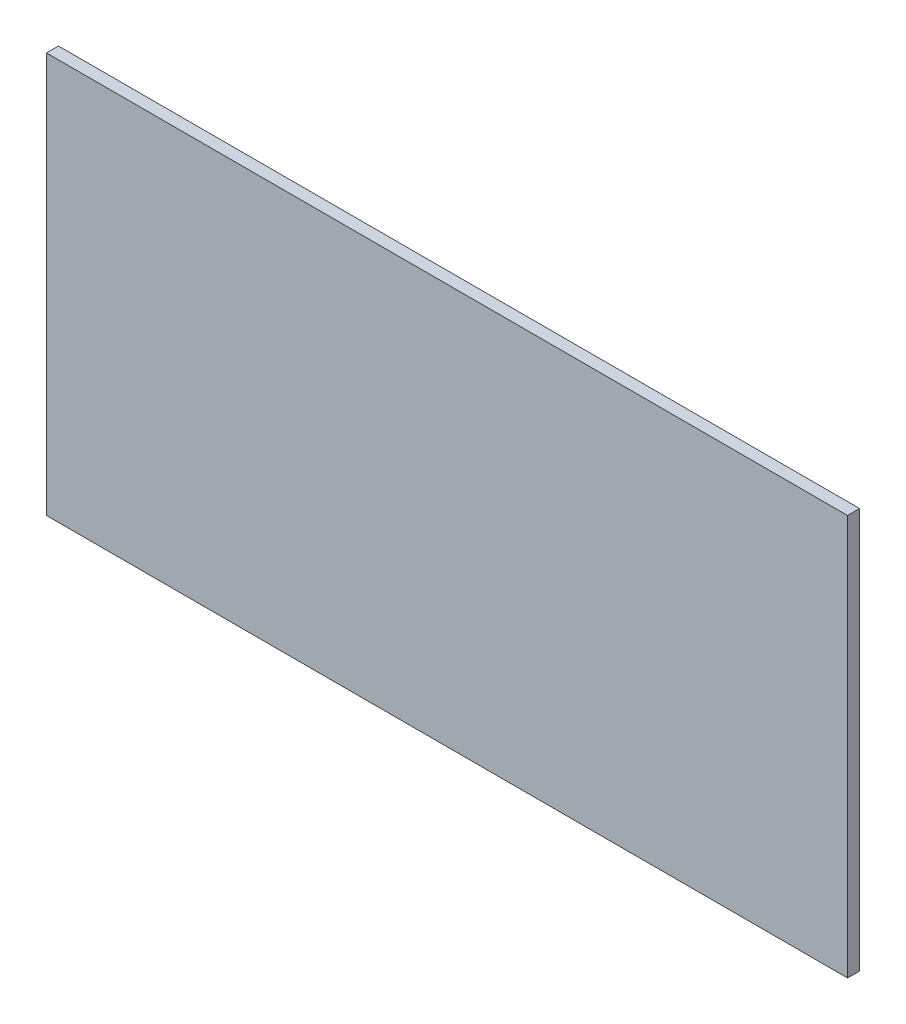
# Autodesk Inventor part: 받침
Saved by Autodesk Inventor 2016 (Build 200138000, 138)
## iProperties
Created: 2024-03-15
Part Number: 받침
Material: 카펫
Document SubType Name: Modeling
Designer: pc
Density: 0.19 g/cm^3
Appearance: 섬세 - 흰색
Author: pc
Autodesk Inventor part; units mm, degrees
ref_plane "YZ Plane" through (0, 0, 0) normal (1, 0, 0) x (0, 1, 0)
ref_plane "XZ Plane" through (0, 0, 0) normal (0, 1, 0) x (-1, 0, 0)
ref_plane "XY Plane" through (0, 0, 0) normal (0, 0, 1) x (1, 0, 0)
sketch "스케치1" plane through (0, 0, 0) normal (0, 0, 1) x (1, 0, 0)
  line L0 (2863.1017, -1431.5508) -> (2663.1017, -1431.5508)
  line L1 (2663.1017, -1431.5508) -> (2663.1017, -1331.5508)
  line L2 (2663.1017, -1331.5508) -> (2863.1017, -1331.5508)
  line L3 (2863.1017, -1331.5508) -> (2863.1017, -1431.5508)
  line L4 (2863.1017, -1431.5508) -> (2663.1017, -1331.5508) construction
  line L5 (0, 0) -> (2863.1017, -1331.5508) construction
  point P0 (0, 0)
  dimension "d0" = 200
  dimension "d1" = 100
  constraints: 12 end point, 3 point on line, 2 parallel, 1 horizontal, 1 perpendicular
  measures "d0" distance of L0.start L0.end
  measures "d1" distance of L0.end L1.end
extrude "돌출1" add sketch "스케치1" along normal blind 3
sketch "스케치2" plane through (0, 0, 3) normal (0, 0, 1) x (1, 0, 0)
  point P0 (0, 0)
sketch "스케치3" plane through (0, 0, 3) normal (0, 0, 1) x (1, 0, 0)
  point P0 (0, 0)
sketch "스케치4" plane through (0, 0, 3) normal (0, 0, 1) x (1, 0, 0)
  point P0 (0, 0)
